Autodesk Fusion 360 part; units mm, degrees
(part 2 of 3)
sketch "Sketch5" plane through (0, 5.5, 0) normal (0, 1, 0) x (-1, 0, 0)
  line L0 (0, 36) -> (-36, 36)
  line L1 (-36, 36) -> (-36, 0)
  line L2 (-36, 0) -> (0, 0)
  line L3 (0, 0) -> (0, 36)
  circle A0 centre (-33.25, 2.75) radius 1.5
  circle A1 centre (-33.25, 33.25) radius 1.5
  circle A2 centre (-2.75, 2.75) radius 1.5
  circle A3 centre (-2.75, 33.25) radius 1.5
  line L4 (-31, 32) -> (-31, 35)
  line L5 (-31, 35) -> (-29, 35)
  line L6 (-29, 35) -> (-29, 32)
  line L7 (-29, 32) -> (-31, 32)
  line L8 (-31, 27.5714) -> (-31, 30.5714)
  line L9 (-31, 30.5714) -> (-29, 30.5714)
  line L10 (-29, 30.5714) -> (-29, 27.5714)
  line L11 (-29, 27.5714) -> (-31, 27.5714)
  line L12 (-31, 23.1429) -> (-31, 26.1429)
  line L13 (-31, 26.1429) -> (-29, 26.1429)
  line L14 (-29, 26.1429) -> (-29, 23.1429)
  line L15 (-29, 23.1429) -> (-31, 23.1429)
  line L16 (-31, 18.7143) -> (-31, 21.7143)
  line L17 (-31, 21.7143) -> (-29, 21.7143)
  line L18 (-29, 21.7143) -> (-29, 18.7143)
  line L19 (-29, 18.7143) -> (-31, 18.7143)
  line L20 (-31, 14.2857) -> (-31, 17.2857)
  line L21 (-31, 17.2857) -> (-29, 17.2857)
  line L22 (-29, 17.2857) -> (-29, 14.2857)
  line L23 (-29, 14.2857) -> (-31, 14.2857)
  line L24 (-31, 9.8571) -> (-31, 12.8571)
  line L25 (-31, 12.8571) -> (-29, 12.8571)
  line L26 (-29, 12.8571) -> (-29, 9.8571)
  line L27 (-29, 9.8571) -> (-31, 9.8571)
  line L28 (-31, 5.4286) -> (-31, 8.4286)
  line L29 (-31, 8.4286) -> (-29, 8.4286)
  line L30 (-29, 8.4286) -> (-29, 5.4286)
  line L31 (-29, 5.4286) -> (-31, 5.4286)
  line L32 (-31, 1) -> (-31, 4)
  line L33 (-31, 4) -> (-29, 4)
  line L34 (-29, 4) -> (-29, 1)
  line L35 (-29, 1) -> (-31, 1)
  line L36 (-27, 32) -> (-27, 35)
  line L37 (-27, 35) -> (-25, 35)
  line L38 (-25, 35) -> (-25, 32)
  line L39 (-25, 32) -> (-27, 32)
  line L40 (-27, 27.5714) -> (-27, 30.5714)
  line L41 (-27, 30.5714) -> (-25, 30.5714)
  line L42 (-25, 30.5714) -> (-25, 27.5714)
  line L43 (-25, 27.5714) -> (-27, 27.5714)
  line L44 (-27, 23.1429) -> (-27, 26.1429)
  line L45 (-27, 26.1429) -> (-25, 26.1429)
  line L46 (-25, 26.1429) -> (-25, 23.1429)
  line L47 (-25, 23.1429) -> (-27, 23.1429)
  line L48 (-27, 18.7143) -> (-27, 21.7143)
  line L49 (-27, 21.7143) -> (-25, 21.7143)
  line L50 (-25, 21.7143) -> (-25, 18.7143)
  line L51 (-25, 18.7143) -> (-27, 18.7143)
  line L52 (-27, 14.2857) -> (-27, 17.2857)
  line L53 (-27, 17.2857) -> (-25, 17.2857)
  line L54 (-25, 17.2857) -> (-25, 14.2857)
  line L55 (-25, 14.2857) -> (-27, 14.2857)
  line L56 (-27, 9.8571) -> (-27, 12.8571)
  line L57 (-27, 12.8571) -> (-25, 12.8571)
  line L58 (-25, 12.8571) -> (-25, 9.8571)
  line L59 (-25, 9.8571) -> (-27, 9.8571)
  line L60 (-27, 5.4286) -> (-27, 8.4286)
  line L61 (-27, 8.4286) -> (-25, 8.4286)
  line L62 (-25, 8.4286) -> (-25, 5.4286)
  line L63 (-25, 5.4286) -> (-27, 5.4286)
  line L64 (-27, 1) -> (-27, 4)
  line L65 (-27, 4) -> (-25, 4)
  line L66 (-25, 4) -> (-25, 1)
  line L67 (-25, 1) -> (-27, 1)
  line L68 (-23, 32) -> (-23, 35)
  line L69 (-23, 35) -> (-21, 35)
  line L70 (-21, 35) -> (-21, 32)
  line L71 (-21, 32) -> (-23, 32)
  line L72 (-23, 27.5714) -> (-23, 30.5714)
  line L73 (-23, 30.5714) -> (-21, 30.5714)
  line L74 (-21, 30.5714) -> (-21, 27.5714)
  line L75 (-21, 27.5714) -> (-23, 27.5714)
  line L76 (-23, 23.1429) -> (-23, 26.1429)
  line L77 (-23, 26.1429) -> (-21, 26.1429)
  line L78 (-21, 26.1429) -> (-21, 23.1429)
  line L79 (-21, 23.1429) -> (-23, 23.1429)
  line L80 (-23, 18.7143) -> (-23, 21.7143)
  line L81 (-23, 21.7143) -> (-21, 21.7143)
  line L82 (-21, 21.7143) -> (-21, 18.7143)
  line L83 (-21, 18.7143) -> (-23, 18.7143)
  line L84 (-23, 14.2857) -> (-23, 17.2857)
  line L85 (-23, 17.2857) -> (-21, 17.2857)
  line L86 (-21, 17.2857) -> (-21, 14.2857)
  line L87 (-21, 14.2857) -> (-23, 14.2857)
  line L88 (-23, 9.8571) -> (-23, 12.8571)
  line L89 (-23, 12.8571) -> (-21, 12.8571)
  line L90 (-21, 12.8571) -> (-21, 9.8571)
  line L91 (-21, 9.8571) -> (-23, 9.8571)
  line L92 (-23, 5.4286) -> (-23, 8.4286)
  line L93 (-23, 8.4286) -> (-21, 8.4286)
  line L94 (-21, 8.4286) -> (-21, 5.4286)
  line L95 (-21, 5.4286) -> (-23, 5.4286)
  line L96 (-23, 1) -> (-23, 4)
  line L97 (-23, 4) -> (-21, 4)
  line L98 (-21, 4) -> (-21, 1)
  line L99 (-21, 1) -> (-23, 1)
  line L100 (-19, 32) -> (-19, 35)
  line L101 (-19, 35) -> (-17, 35)
  line L102 (-17, 35) -> (-17, 32)
  line L103 (-17, 32) -> (-19, 32)
  line L104 (-19, 27.5714) -> (-19, 30.5714)
  line L105 (-19, 30.5714) -> (-17, 30.5714)
  line L106 (-17, 30.5714) -> (-17, 27.5714)
  line L107 (-17, 27.5714) -> (-19, 27.5714)
  line L108 (-19, 23.1429) -> (-19, 26.1429)
  line L109 (-19, 26.1429) -> (-17, 26.1429)
  line L110 (-17, 26.1429) -> (-17, 23.1429)
  line L111 (-17, 23.1429) -> (-19, 23.1429)
  line L112 (-19, 18.7143) -> (-19, 21.7143)
  line L113 (-19, 21.7143) -> (-17, 21.7143)
  line L114 (-17, 21.7143) -> (-17, 18.7143)
  line L115 (-17, 18.7143) -> (-19, 18.7143)
  line L116 (-19, 14.2857) -> (-19, 17.2857)
  line L117 (-19, 17.2857) -> (-17, 17.2857)
  line L118 (-17, 17.2857) -> (-17, 14.2857)
  line L119 (-17, 14.2857) -> (-19, 14.2857)
  line L120 (-19, 9.8571) -> (-19, 12.8571)
  line L121 (-19, 12.8571) -> (-17, 12.8571)
  line L122 (-17, 12.8571) -> (-17, 9.8571)
  line L123 (-17, 9.8571) -> (-19, 9.8571)
  line L124 (-19, 5.4286) -> (-19, 8.4286)
  line L125 (-19, 8.4286) -> (-17, 8.4286)
  line L126 (-17, 8.4286) -> (-17, 5.4286)
  line L127 (-17, 5.4286) -> (-19, 5.4286)
  line L128 (-19, 1) -> (-19, 4)
  line L129 (-19, 4) -> (-17, 4)
  line L130 (-17, 4) -> (-17, 1)
  line L131 (-17, 1) -> (-19, 1)
  line L132 (-15, 32) -> (-15, 35)
  line L133 (-15, 35) -> (-13, 35)
  line L134 (-13, 35) -> (-13, 32)
  line L135 (-13, 32) -> (-15, 32)
  line L136 (-15, 27.5714) -> (-15, 30.5714)
  line L137 (-15, 30.5714) -> (-13, 30.5714)
  line L138 (-13, 30.5714) -> (-13, 27.5714)
  line L139 (-13, 27.5714) -> (-15, 27.5714)
  line L140 (-15, 23.1429) -> (-15, 26.1429)
  line L141 (-15, 26.1429) -> (-13, 26.1429)
  line L142 (-13, 26.1429) -> (-13, 23.1429)
  line L143 (-13, 23.1429) -> (-15, 23.1429)
  line L144 (-15, 18.7143) -> (-15, 21.7143)
  line L145 (-15, 21.7143) -> (-13, 21.7143)
  line L146 (-13, 21.7143) -> (-13, 18.7143)
  line L147 (-13, 18.7143) -> (-15, 18.7143)
  line L148 (-15, 14.2857) -> (-15, 17.2857)
  line L149 (-15, 17.2857) -> (-13, 17.2857)
  line L150 (-13, 17.2857) -> (-13, 14.2857)
  line L151 (-13, 14.2857) -> (-15, 14.2857)
  line L152 (-15, 9.8571) -> (-15, 12.8571)
  line L153 (-15, 12.8571) -> (-13, 12.8571)
  line L154 (-13, 12.8571) -> (-13, 9.8571)
  line L155 (-13, 9.8571) -> (-15, 9.8571)
  line L156 (-15, 5.4286) -> (-15, 8.4286)
  line L157 (-15, 8.4286) -> (-13, 8.4286)
  line L158 (-13, 8.4286) -> (-13, 5.4286)
  line L159 (-13, 5.4286) -> (-15, 5.4286)
  line L160 (-15, 1) -> (-15, 4)
  line L161 (-15, 4) -> (-13, 4)
  line L162 (-13, 4) -> (-13, 1)
  line L163 (-13, 1) -> (-15, 1)
  line L164 (-11, 32) -> (-11, 35)
  line L165 (-11, 35) -> (-9, 35)
  line L166 (-9, 35) -> (-9, 32)
  line L167 (-9, 32) -> (-11, 32)
  line L168 (-11, 27.5714) -> (-11, 30.5714)
  line L169 (-11, 30.5714) -> (-9, 30.5714)
  line L170 (-9, 30.5714) -> (-9, 27.5714)
  line L171 (-9, 27.5714) -> (-11, 27.5714)
  line L172 (-11, 23.1429) -> (-11, 26.1429)
  line L173 (-11, 26.1429) -> (-9, 26.1429)
  line L174 (-9, 26.1429) -> (-9, 23.1429)
  line L175 (-9, 23.1429) -> (-11, 23.1429)
  line L176 (-11, 18.7143) -> (-11, 21.7143)
  line L177 (-11, 21.7143) -> (-9, 21.7143)
  line L178 (-9, 21.7143) -> (-9, 18.7143)
  line L179 (-9, 18.7143) -> (-11, 18.7143)
  line L180 (-11, 14.2857) -> (-11, 17.2857)
  line L181 (-11, 17.2857) -> (-9, 17.2857)
  line L182 (-9, 17.2857) -> (-9, 14.2857)
  line L183 (-9, 14.2857) -> (-11, 14.2857)
  line L184 (-11, 9.8571) -> (-11, 12.8571)
  line L185 (-11, 12.8571) -> (-9, 12.8571)
  line L186 (-9, 12.8571) -> (-9, 9.8571)
  line L187 (-9, 9.8571) -> (-11, 9.8571)
  line L188 (-11, 5.4286) -> (-11, 8.4286)
  line L189 (-11, 8.4286) -> (-9, 8.4286)
  line L190 (-9, 8.4286) -> (-9, 5.4286)
  line L191 (-9, 5.4286) -> (-11, 5.4286)
  line L192 (-11, 1) -> (-11, 4)
  line L193 (-11, 4) -> (-9, 4)
  line L194 (-9, 4) -> (-9, 1)
  line L195 (-9, 1) -> (-11, 1)
  line L196 (-7, 32) -> (-7, 35)
  line L197 (-7, 35) -> (-5, 35)
  line L198 (-5, 35) -> (-5, 32)
  line L199 (-5, 32) -> (-7, 32)
  line L200 (-7, 27.5714) -> (-7, 30.5714)
  line L201 (-7, 30.5714) -> (-5, 30.5714)
  line L202 (-5, 30.5714) -> (-5, 27.5714)
  line L203 (-5, 27.5714) -> (-7, 27.5714)
  line L204 (-7, 23.1429) -> (-7, 26.1429)
  line L205 (-7, 26.1429) -> (-5, 26.1429)
  line L206 (-5, 26.1429) -> (-5, 23.1429)
  line L207 (-5, 23.1429) -> (-7, 23.1429)
  line L208 (-7, 18.7143) -> (-7, 21.7143)
  line L209 (-7, 21.7143) -> (-5, 21.7143)
  line L210 (-5, 21.7143) -> (-5, 18.7143)
  line L211 (-5, 18.7143) -> (-7, 18.7143)
  line L212 (-7, 14.2857) -> (-7, 17.2857)
  line L213 (-7, 17.2857) -> (-5, 17.2857)
  line L214 (-5, 17.2857) -> (-5, 14.2857)
  line L215 (-5, 14.2857) -> (-7, 14.2857)
  line L216 (-7, 9.8571) -> (-7, 12.8571)
  line L217 (-7, 12.8571) -> (-5, 12.8571)
  line L218 (-5, 12.8571) -> (-5, 9.8571)
  line L219 (-5, 9.8571) -> (-7, 9.8571)
  line L220 (-7, 5.4286) -> (-7, 8.4286)
  line L221 (-7, 8.4286) -> (-5, 8.4286)
  line L222 (-5, 8.4286) -> (-5, 5.4286)
  line L223 (-5, 5.4286) -> (-7, 5.4286)
  line L224 (-7, 1) -> (-7, 4)
  line L225 (-7, 4) -> (-5, 4)
  line L226 (-5, 4) -> (-5, 1)
  line L227 (-5, 1) -> (-7, 1)
  line L228 (-4, 31) -> (0.3, 31)
  line L229 (0.3, 31) -> (-4, 31)
  line L230 (-4, 31) -> (-4, 5)
  line L231 (-4, 5) -> (0.5, 5)
  constraint perpendicular L3 L228
  constraint perpendicular L219 L230
  constraint perpendicular L3 L231
extrude "Extrude5" cut sketch "Sketch5" against normal blind 15 contours L3 L228 L229 L230 L231
sketch "Sketch6" plane through (0, 5.5, 0) normal (0, 1, 0) x (-1, 0, 0)
  line L0 (-7, 1) -> (-7, 4)
  line L1 (-7, 4) -> (-5, 4)
  line L2 (-5, 4) -> (-5, 1)
  line L3 (-5, 1) -> (-7, 1)
  line L4 (-7, 5.4286) -> (-7, 8.4286)
  line L5 (-7, 8.4286) -> (-5, 8.4286)
  line L6 (-5, 8.4286) -> (-5, 5.4286)
  line L7 (-5, 5.4286) -> (-7, 5.4286)
  line L8 (-7, 9.8571) -> (-7, 12.8571)
  line L9 (-7, 12.8571) -> (-5, 12.8571)
  line L10 (-5, 12.8571) -> (-5, 9.8571)
  line L11 (-5, 9.8571) -> (-7, 9.8571)
  line L12 (-7, 14.2857) -> (-7, 17.2857)
  line L13 (-7, 17.2857) -> (-5, 17.2857)
  line L14 (-5, 17.2857) -> (-5, 14.2857)
  line L15 (-5, 14.2857) -> (-7, 14.2857)
  line L16 (-7, 18.7143) -> (-7, 21.7143)
  line L17 (-7, 21.7143) -> (-5, 21.7143)
  line L18 (-5, 21.7143) -> (-5, 18.7143)
  line L19 (-5, 18.7143) -> (-7, 18.7143)
  line L20 (-7, 23.1429) -> (-7, 26.1429)
  line L21 (-7, 26.1429) -> (-5, 26.1429)
  line L22 (-5, 26.1429) -> (-5, 23.1429)
  line L23 (-5, 23.1429) -> (-7, 23.1429)
  line L24 (-7, 27.5714) -> (-7, 30.5714)
  line L25 (-7, 30.5714) -> (-5, 30.5714)
  line L26 (-5, 30.5714) -> (-5, 27.5714)
  line L27 (-5, 27.5714) -> (-7, 27.5714)
  line L28 (-7, 32) -> (-7, 35)
  line L29 (-7, 35) -> (-5, 35)
  line L30 (-5, 35) -> (-5, 32)
  line L31 (-5, 32) -> (-7, 32)
  line L32 (-11, 1) -> (-11, 4)
  line L33 (-11, 4) -> (-9, 4)
  line L34 (-9, 4) -> (-9, 1)
  line L35 (-9, 1) -> (-11, 1)
  line L36 (-11, 5.4286) -> (-11, 8.4286)
  line L37 (-11, 8.4286) -> (-9, 8.4286)
  line L38 (-9, 8.4286) -> (-9, 5.4286)
  line L39 (-9, 5.4286) -> (-11, 5.4286)
  line L40 (-11, 9.8571) -> (-11, 12.8571)
  line L41 (-11, 12.8571) -> (-9, 12.8571)
  line L42 (-9, 12.8571) -> (-9, 9.8571)
  line L43 (-9, 9.8571) -> (-11, 9.8571)
  line L44 (-11, 14.2857) -> (-11, 17.2857)
  line L45 (-11, 17.2857) -> (-9, 17.2857)
  line L46 (-9, 17.2857) -> (-9, 14.2857)
  line L47 (-9, 14.2857) -> (-11, 14.2857)
  line L48 (-11, 18.7143) -> (-11, 21.7143)
  line L49 (-11, 21.7143) -> (-9, 21.7143)
  line L50 (-9, 21.7143) -> (-9, 18.7143)
  line L51 (-9, 18.7143) -> (-11, 18.7143)
  line L52 (-11, 23.1429) -> (-11, 26.1429)
  line L53 (-11, 26.1429) -> (-9, 26.1429)
  line L54 (-9, 26.1429) -> (-9, 23.1429)
  line L55 (-9, 23.1429) -> (-11, 23.1429)
  line L56 (-11, 27.5714) -> (-11, 30.5714)
  line L57 (-11, 30.5714) -> (-9, 30.5714)
  line L58 (-9, 30.5714) -> (-9, 27.5714)
  line L59 (-9, 27.5714) -> (-11, 27.5714)
  line L60 (-11, 32) -> (-11, 35)
  line L61 (-11, 35) -> (-9, 35)
  line L62 (-9, 35) -> (-9, 32)
  line L63 (-9, 32) -> (-11, 32)
  line L64 (-15, 1) -> (-15, 4)
  line L65 (-15, 4) -> (-13, 4)
  line L66 (-13, 4) -> (-13, 1)
  line L67 (-13, 1) -> (-15, 1)
  line L68 (-15, 5.4286) -> (-15, 8.4286)
  line L69 (-15, 8.4286) -> (-13, 8.4286)
  line L70 (-13, 8.4286) -> (-13, 5.4286)
  line L71 (-13, 5.4286) -> (-15, 5.4286)
  line L72 (-15, 9.8571) -> (-15, 12.8571)
  line L73 (-15, 12.8571) -> (-13, 12.8571)
  line L74 (-13, 12.8571) -> (-13, 9.8571)
  line L75 (-13, 9.8571) -> (-15, 9.8571)
  line L76 (-15, 14.2857) -> (-15, 17.2857)
  line L77 (-15, 17.2857) -> (-13, 17.2857)
  line L78 (-13, 17.2857) -> (-13, 14.2857)
  line L79 (-13, 14.2857) -> (-15, 14.2857)
  line L80 (-15, 18.7143) -> (-15, 21.7143)
  line L81 (-15, 21.7143) -> (-13, 21.7143)
  line L82 (-13, 21.7143) -> (-13, 18.7143)
  line L83 (-13, 18.7143) -> (-15, 18.7143)
  line L84 (-15, 23.1429) -> (-15, 26.1429)
  line L85 (-15, 26.1429) -> (-13, 26.1429)
  line L86 (-13, 26.1429) -> (-13, 23.1429)
  line L87 (-13, 23.1429) -> (-15, 23.1429)
  line L88 (-15, 27.5714) -> (-15, 30.5714)
  line L89 (-15, 30.5714) -> (-13, 30.5714)
  line L90 (-13, 30.5714) -> (-13, 27.5714)
  line L91 (-13, 27.5714) -> (-15, 27.5714)
  line L92 (-15, 32) -> (-15, 35)
  line L93 (-15, 35) -> (-13, 35)
  line L94 (-13, 35) -> (-13, 32)
  line L95 (-13, 32) -> (-15, 32)
  line L96 (-19, 1) -> (-19, 4)
  line L97 (-19, 4) -> (-17, 4)
  line L98 (-17, 4) -> (-17, 1)
  line L99 (-17, 1) -> (-19, 1)
  line L100 (-19, 5.4286) -> (-19, 8.4286)
  line L101 (-19, 8.4286) -> (-17, 8.4286)
  line L102 (-17, 8.4286) -> (-17, 5.4286)
  line L103 (-17, 5.4286) -> (-19, 5.4286)
  line L104 (-19, 9.8571) -> (-19, 12.8571)
  line L105 (-19, 12.8571) -> (-17, 12.8571)
  line L106 (-17, 12.8571) -> (-17, 9.8571)
  line L107 (-17, 9.8571) -> (-19, 9.8571)
  line L108 (-19, 14.2857) -> (-19, 17.2857)
  line L109 (-19, 17.2857) -> (-17, 17.2857)
  line L110 (-17, 17.2857) -> (-17, 14.2857)
  line L111 (-17, 14.2857) -> (-19, 14.2857)
  line L112 (-19, 18.7143) -> (-19, 21.7143)
  line L113 (-19, 21.7143) -> (-17, 21.7143)
  line L114 (-17, 21.7143) -> (-17, 18.7143)
  line L115 (-17, 18.7143) -> (-19, 18.7143)
  line L116 (-19, 23.1429) -> (-19, 26.1429)
  line L117 (-19, 26.1429) -> (-17, 26.1429)
  line L118 (-17, 26.1429) -> (-17, 23.1429)
  line L119 (-17, 23.1429) -> (-19, 23.1429)
  line L120 (-19, 27.5714) -> (-19, 30.5714)
  line L121 (-19, 30.5714) -> (-17, 30.5714)
  line L122 (-17, 30.5714) -> (-17, 27.5714)
  line L123 (-17, 27.5714) -> (-19, 27.5714)
  line L124 (-19, 32) -> (-19, 35)
  line L125 (-19, 35) -> (-17, 35)
  line L126 (-17, 35) -> (-17, 32)
  line L127 (-17, 32) -> (-19, 32)
  line L128 (-23, 1) -> (-23, 4)
  line L129 (-23, 4) -> (-21, 4)
  line L130 (-21, 4) -> (-21, 1)
  line L131 (-21, 1) -> (-23, 1)
  line L132 (-23, 5.4286) -> (-23, 8.4286)
  line L133 (-23, 8.4286) -> (-21, 8.4286)
  line L134 (-21, 8.4286) -> (-21, 5.4286)
  line L135 (-21, 5.4286) -> (-23, 5.4286)
  line L136 (-23, 9.8571) -> (-23, 12.8571)
  line L137 (-23, 12.8571) -> (-21, 12.8571)
  line L138 (-21, 12.8571) -> (-21, 9.8571)
  line L139 (-21, 9.8571) -> (-23, 9.8571)
  line L140 (-23, 14.2857) -> (-23, 17.2857)
  line L141 (-23, 17.2857) -> (-21, 17.2857)
  line L142 (-21, 17.2857) -> (-21, 14.2857)
  line L143 (-21, 14.2857) -> (-23, 14.2857)
  line L144 (-23, 18.7143) -> (-23, 21.7143)
  line L145 (-23, 21.7143) -> (-21, 21.7143)
  line L146 (-21, 21.7143) -> (-21, 18.7143)
  line L147 (-21, 18.7143) -> (-23, 18.7143)
  line L148 (-23, 23.1429) -> (-23, 26.1429)
  line L149 (-23, 26.1429) -> (-21, 26.1429)
  line L150 (-21, 26.1429) -> (-21, 23.1429)
  line L151 (-21, 23.1429) -> (-23, 23.1429)
  line L152 (-23, 27.5714) -> (-23, 30.5714)
  line L153 (-23, 30.5714) -> (-21, 30.5714)
  line L154 (-21, 30.5714) -> (-21, 27.5714)
  line L155 (-21, 27.5714) -> (-23, 27.5714)
  line L156 (-23, 32) -> (-23, 35)
  line L157 (-23, 35) -> (-21, 35)
  line L158 (-21, 35) -> (-21, 32)
  line L159 (-21, 32) -> (-23, 32)
  line L160 (-27, 1) -> (-27, 4)
  line L161 (-27, 4) -> (-25, 4)
  line L162 (-25, 4) -> (-25, 1)
  line L163 (-25, 1) -> (-27, 1)
  line L164 (-27, 5.4286) -> (-27, 8.4286)
  line L165 (-27, 8.4286) -> (-25, 8.4286)
  line L166 (-25, 8.4286) -> (-25, 5.4286)
  line L167 (-25, 5.4286) -> (-27, 5.4286)
  line L168 (-27, 9.8571) -> (-27, 12.8571)
  line L169 (-27, 12.8571) -> (-25, 12.8571)
  line L170 (-25, 12.8571) -> (-25, 9.8571)
  line L171 (-25, 9.8571) -> (-27, 9.8571)
  line L172 (-27, 14.2857) -> (-27, 17.2857)
  line L173 (-27, 17.2857) -> (-25, 17.2857)
  line L174 (-25, 17.2857) -> (-25, 14.2857)
  line L175 (-25, 14.2857) -> (-27, 14.2857)
  line L176 (-27, 18.7143) -> (-27, 21.7143)
  line L177 (-27, 21.7143) -> (-25, 21.7143)
  line L178 (-25, 21.7143) -> (-25, 18.7143)
  line L179 (-25, 18.7143) -> (-27, 18.7143)
  line L180 (-27, 23.1429) -> (-27, 26.1429)
  line L181 (-27, 26.1429) -> (-25, 26.1429)
  line L182 (-25, 26.1429) -> (-25, 23.1429)
  line L183 (-25, 23.1429) -> (-27, 23.1429)
  line L184 (-27, 27.5714) -> (-27, 30.5714)
  line L185 (-27, 30.5714) -> (-25, 30.5714)
  line L186 (-25, 30.5714) -> (-25, 27.5714)
  line L187 (-25, 27.5714) -> (-27, 27.5714)
  line L188 (-27, 32) -> (-27, 35)
  line L189 (-27, 35) -> (-25, 35)
  line L190 (-25, 35) -> (-25, 32)
  line L191 (-25, 32) -> (-27, 32)
  line L192 (-31, 1) -> (-31, 4)
  line L193 (-31, 4) -> (-29, 4)
  line L194 (-29, 4) -> (-29, 1)
  line L195 (-29, 1) -> (-31, 1)
  line L196 (-31, 5.4286) -> (-31, 8.4286)
  line L197 (-31, 8.4286) -> (-29, 8.4286)
  line L198 (-29, 8.4286) -> (-29, 5.4286)
  line L199 (-29, 5.4286) -> (-31, 5.4286)
  line L200 (-31, 9.8571) -> (-31, 12.8571)
  line L201 (-31, 12.8571) -> (-29, 12.8571)
  line L202 (-29, 12.8571) -> (-29, 9.8571)
  line L203 (-29, 9.8571) -> (-31, 9.8571)
  line L204 (-31, 14.2857) -> (-31, 17.2857)
  line L205 (-31, 17.2857) -> (-29, 17.2857)
  line L206 (-29, 17.2857) -> (-29, 14.2857)
  line L207 (-29, 14.2857) -> (-31, 14.2857)
  line L208 (-31, 18.7143) -> (-31, 21.7143)
  line L209 (-31, 21.7143) -> (-29, 21.7143)
  line L210 (-29, 21.7143) -> (-29, 18.7143)
  line L211 (-29, 18.7143) -> (-31, 18.7143)
  line L212 (-31, 23.1429) -> (-31, 26.1429)
  line L213 (-31, 26.1429) -> (-29, 26.1429)
  line L214 (-29, 26.1429) -> (-29, 23.1429)
  line L215 (-29, 23.1429) -> (-31, 23.1429)
  line L216 (-31, 27.5714) -> (-31, 30.5714)
  line L217 (-31, 30.5714) -> (-29, 30.5714)
  line L218 (-29, 30.5714) -> (-29, 27.5714)
  line L219 (-29, 27.5714) -> (-31, 27.5714)
  line L220 (-31, 32) -> (-31, 35)
  line L221 (-31, 35) -> (-29, 35)
  line L222 (-29, 35) -> (-29, 32)
  line L223 (-29, 32) -> (-31, 32)
  circle A0 centre (-2.75, 33.25) radius 1.5
  circle A1 centre (-2.75, 2.75) radius 1.5
  circle A2 centre (-33.25, 33.25) radius 1.5
  circle A3 centre (-33.25, 2.75) radius 1.5
  line L224 (-4, 31) -> (0, 31)
  line L225 (0, 31) -> (0, 36)
  line L226 (0, 36) -> (-36, 36)
  line L227 (-36, 36) -> (-36, 0)
  line L228 (-36, 0) -> (0, 0)
  line L229 (0, 0) -> (0, 5)
  line L230 (0, 5) -> (-4, 5)
  line L231 (-4, 5) -> (-4, 31)
  line L232 (-36, 31) -> (-32, 31)
  line L233 (-32, 31) -> (-32, 5)
  line L234 (-32, 5) -> (-36, 5)
  constraint coincident L227 L232.start
  constraint perpendicular L227 L232
  constraint perpendicular L199 L233
  constraint coincident L227 L234.end
  constraint perpendicular L227 L234
extrude "Extrude6" cut sketch "Sketch6" against normal blind 15 contours L227 L232 L233 L234
sketch "Sketch7" plane through (0, 0, 36) normal (0, 0, 1) x (-1, 0, 0)
  line L0 (0, 0) -> (-36, 0)
  line L1 (-36, 0) -> (-36, -5.5)
  line L2 (-36, -5.5) -> (0, -5.5)
  line L3 (0, -5.5) -> (0, 0)
  circle A0 centre (-18, -2.75) radius 2.5
  dimension "d32" = 5
  measures "d32" diameter of A0
extrude "Extrude7" add sketch "Sketch7" along normal blind 3 contours A0
sketch "Sketch8" plane through (0, 0, 0) normal (0, -1, 0) x (1, 0, 0)
  line L0 (32, 31) -> (36, 31)
  line L1 (36, 31) -> (36, 36)
  line L2 (36, 36) -> (0, 36)
  line L3 (0, 36) -> (0, 31)
  line L4 (0, 31) -> (4, 31)
  line L5 (4, 31) -> (4, 5)
  line L6 (4, 5) -> (0, 5)
  line L7 (0, 5) -> (0, 0)
  line L8 (0, 0) -> (36, 0)
  line L9 (36, 0) -> (36, 5)
  line L10 (36, 5) -> (32, 5)
  line L11 (32, 5) -> (32, 31)
  circle A0 centre (33.25, 2.75) radius 1.5
  circle A1 centre (33.25, 33.25) radius 1.5
  circle A2 centre (2.75, 2.75) radius 1.5
  circle A3 centre (2.75, 33.25) radius 1.5
  line L12 (31, 18) -> (29, 18)
  line L13 (29, 18) -> (29, 28)
  line L14 (29, 28) -> (31, 28)
  line L15 (31, 28) -> (31, 18)
  line L16 (29.2903, 27.5521) -> (30.7537, 27.5521)
  line L17 (30.7537, 27.5521) -> (30.7537, 25.0331)
  line L18 (30.7537, 25.0331) -> (29.2903, 25.0331)
  line L19 (29.2903, 25.0331) -> (29.2903, 27.5521)
  line L20 (29.2903, 24.3827) -> (30.7537, 24.3827)
  line L21 (30.7537, 24.3827) -> (30.7537, 21.7556)
  line L22 (30.7537, 21.7556) -> (29.2903, 21.7556)
  line L23 (29.2903, 21.7556) -> (29.2903, 24.3827)
  line L24 (29.2903, 21.0379) -> (30.7537, 21.0379)
  line L25 (30.7537, 21.0379) -> (30.7537, 18.3132)
  line L26 (30.7537, 18.3132) -> (29.2903, 18.3132)
  line L27 (29.2903, 18.3132) -> (29.2903, 21.0379)
  constraint horizontal L12
  constraint vertical L13
  constraint horizontal L14
  constraint vertical L15
  constraint horizontal L16
  constraint vertical L17
  constraint horizontal L18
  constraint vertical L19
  constraint horizontal L20
  constraint vertical L21
  constraint horizontal L22
  constraint vertical L23
  constraint horizontal L24
  constraint vertical L25
  constraint horizontal L26
  constraint vertical L27
extrude "Extrude8" add sketch "Sketch8" along normal blind 1 contours L16 L17 L18 L19 | L20 L21 L22 L23 | L24 L25 L26 L27
sketch "Sketch9" plane through (32, 0, 0) normal (1, 0, 0) x (0, 1, 0)
  line L0 (0, 31) -> (0, 5)
  line L1 (0, 5) -> (5.5, 5)
  line L2 (5.5, 5) -> (5.5, 31)
  line L3 (5.5, 31) -> (0, 31)
  line L4 (2, 12.9249) -> (3.5, 12.9249)
  line L5 (3.5, 12.9249) -> (3.5, 10)
  line L6 (3.5, 10) -> (2, 10)
  line L7 (2, 10) -> (2, 12.9249)
  constraint horizontal L4
  constraint vertical L5
  constraint horizontal L6
  constraint vertical L7
extrude "Extrude9" add sketch "Sketch9" along normal blind 1 contours L4 L5 L6 L7
sketch "Sketch10" plane through (0, 0, 0) normal (0, -1, 0) x (1, 0, 0)
  line L0 (29.2903, 25.0331) -> (29.2903, 27.5521)
  line L1 (29.2903, 27.5521) -> (30.7537, 27.5521)
  line L2 (30.7537, 27.5521) -> (30.7537, 25.0331)
  line L3 (30.7537, 25.0331) -> (29.2903, 25.0331)
  line L4 (29.2903, 21.7556) -> (29.2903, 24.3827)
  line L5 (29.2903, 24.3827) -> (30.7537, 24.3827)
  line L6 (30.7537, 24.3827) -> (30.7537, 21.7556)
  line L7 (30.7537, 21.7556) -> (29.2903, 21.7556)
  line L8 (29.2903, 18.3132) -> (29.2903, 21.0379)
  line L9 (29.2903, 21.0379) -> (30.7537, 21.0379)
  line L10 (30.7537, 21.0379) -> (30.7537, 18.3132)
  line L11 (30.7537, 18.3132) -> (29.2903, 18.3132)
  line L12 (32, 31) -> (36, 31)
  line L13 (36, 31) -> (36, 36)
  line L14 (36, 36) -> (0, 36)
  line L15 (0, 36) -> (0, 31)
  line L16 (0, 31) -> (4, 31)
  line L17 (4, 31) -> (4, 5)
  line L18 (4, 5) -> (0, 5)
  line L19 (0, 5) -> (0, 0)
  line L20 (0, 0) -> (36, 0)
  line L21 (36, 0) -> (36, 5)
  line L22 (36, 5) -> (32, 5)
  line L23 (32, 5) -> (32, 31)
  circle A0 centre (33.25, 2.75) radius 1.5
  circle A1 centre (33.25, 33.25) radius 1.5
  circle A2 centre (2.75, 2.75) radius 1.5
  circle A3 centre (2.75, 33.25) radius 1.5
  line L24 (5.0897, 18.3132) -> (12, 18.3132)
  line L25 (12, 18.3132) -> (12, 11)
  line L26 (12, 11) -> (5.0897, 11)
  line L27 (5.0897, 11) -> (5.0897, 18.3132)
  constraint horizontal L24
  constraint vertical L25
  constraint horizontal L26
  constraint vertical L27
extrude "Extrude10" add sketch "Sketch10" along normal blind 1 contours L24 L25 L26 L27
sketch "Sketch11" plane through (0, 0, 0) normal (0, -1, 0) x (1, 0, 0)
  circle A0 centre (2.75, 33.25) radius 1.5
  circle A1 centre (2.75, 2.75) radius 1.5
  circle A2 centre (33.25, 33.25) radius 1.5
  circle A3 centre (33.25, 2.75) radius 1.5
  line L0 (32, 31) -> (36, 31)
  line L1 (36, 31) -> (36, 36)
  line L2 (36, 36) -> (0, 36)
  line L3 (0, 36) -> (0, 31)
  line L4 (0, 31) -> (4, 31)
  line L5 (4, 31) -> (4, 5)
  line L6 (4, 5) -> (0, 5)
  line L7 (0, 5) -> (0, 0)
  line L8 (0, 0) -> (36, 0)
  line L9 (36, 0) -> (36, 5)
  line L10 (36, 5) -> (32, 5)
  line L11 (32, 5) -> (32, 31)
  line L12 (29.2903, 18.3132) -> (29.2903, 21.0379)
  line L13 (29.2903, 21.0379) -> (30.7537, 21.0379)
  line L14 (30.7537, 21.0379) -> (30.7537, 18.3132)
  line L15 (30.7537, 18.3132) -> (29.2903, 18.3132)
  line L16 (29.2903, 21.7556) -> (29.2903, 24.3827)
  line L17 (29.2903, 24.3827) -> (30.7537, 24.3827)
  line L18 (30.7537, 24.3827) -> (30.7537, 21.7556)
  line L19 (30.7537, 21.7556) -> (29.2903, 21.7556)
  line L20 (29.2903, 25.0331) -> (29.2903, 27.5521)
  line L21 (29.2903, 27.5521) -> (30.7537, 27.5521)
  line L22 (30.7537, 27.5521) -> (30.7537, 25.0331)
  line L23 (30.7537, 25.0331) -> (29.2903, 25.0331)
  line L24 (5.0897, 11) -> (5.0897, 18.3132)
  line L25 (5.0897, 18.3132) -> (12, 18.3132)
  line L26 (12, 18.3132) -> (12, 11)
  line L27 (12, 11) -> (5.0897, 11)
  line L28 (13, 0) -> (23, 0)
  line L29 (23, 0) -> (23, 4.9683)
  line L30 (23, 4.9683) -> (13, 4.9683)
  line L31 (13, 4.9683) -> (13, 0)
  constraint horizontal L28
  constraint vertical L29
  constraint horizontal L30
  constraint vertical L31
  constraint coincident L8 L28.start
extrude "Extrude11" add sketch "Sketch11" along normal blind 1 contours L8 L28 L29 L30 L31
sketch "Sketch12" plane through (0, 0, 0) normal (0, 0, -1) x (1, 0, 0)
  line L0 (13, 0) -> (0, 0)
  line L1 (0, 0) -> (0, -5.5)
  line L2 (0, -5.5) -> (36, -5.5)
  line L3 (36, -5.5) -> (36, 0)
  line L4 (36, 0) -> (23, 0)
  line L5 (23, 0) -> (23, 1)
  line L6 (23, 1) -> (13, 1)
  line L7 (13, 1) -> (13, 0)
  line L8 (22.621, -1.0763) -> (13.4121, -1.0763)
  line L9 (13.4121, -1.0763) -> (13.4121, 0.5912)
  line L10 (13.4121, 0.5912) -> (22.621, 0.5912)
  line L11 (22.621, 0.5912) -> (22.621, -1.0763)
  constraint horizontal L8
  constraint vertical L9
  constraint horizontal L10
  constraint vertical L11
extrude "Extrude12" cut sketch "Sketch12" against normal blind 1 contours L8 L9 L10 L11
sketch "Sketch13" plane through (0, 5.5, 0) normal (0, 1, 0) x (-1, 0, 0)
  line L0 (-36, 31) -> (-32, 31)
  line L1 (-32, 31) -> (-32, 5)
  line L2 (-32, 5) -> (-36, 5)
  line L3 (-36, 5) -> (-36, 0)
  line L4 (-36, 0) -> (0, 0)
  line L5 (0, 0) -> (0, 5)
  line L6 (0, 5) -> (-4, 5)
  line L7 (-4, 5) -> (-4, 31)
  line L8 (-4, 31) -> (0, 31)
  line L9 (0, 31) -> (0, 36)
  line L10 (0, 36) -> (-36, 36)
  line L11 (-36, 36) -> (-36, 31)
  circle A0 centre (-33.25, 2.75) radius 1.5
  circle A1 centre (-33.25, 33.25) radius 1.5
  circle A2 centre (-2.75, 2.75) radius 1.5
  circle A3 centre (-2.75, 33.25) radius 1.5
  line L12 (-31, 32) -> (-31, 35)
  line L13 (-31, 35) -> (-29, 35)
  line L14 (-29, 35) -> (-29, 32)
  line L15 (-29, 32) -> (-31, 32)
  line L16 (-31, 27.5714) -> (-31, 30.5714)
  line L17 (-31, 30.5714) -> (-29, 30.5714)
  line L18 (-29, 30.5714) -> (-29, 27.5714)
  line L19 (-29, 27.5714) -> (-31, 27.5714)
  line L20 (-31, 23.1429) -> (-31, 26.1429)
  line L21 (-31, 26.1429) -> (-29, 26.1429)
  line L22 (-29, 26.1429) -> (-29, 23.1429)
  line L23 (-29, 23.1429) -> (-31, 23.1429)
  line L24 (-31, 18.7143) -> (-31, 21.7143)
  line L25 (-31, 21.7143) -> (-29, 21.7143)
  line L26 (-29, 21.7143) -> (-29, 18.7143)
  line L27 (-29, 18.7143) -> (-31, 18.7143)
  line L28 (-31, 14.2857) -> (-31, 17.2857)
  line L29 (-31, 17.2857) -> (-29, 17.2857)
  line L30 (-29, 17.2857) -> (-29, 14.2857)
  line L31 (-29, 14.2857) -> (-31, 14.2857)
  line L32 (-31, 9.8571) -> (-31, 12.8571)
  line L33 (-31, 12.8571) -> (-29, 12.8571)
  line L34 (-29, 12.8571) -> (-29, 9.8571)
  line L35 (-29, 9.8571) -> (-31, 9.8571)
  line L36 (-31, 5.4286) -> (-31, 8.4286)
  line L37 (-31, 8.4286) -> (-29, 8.4286)
  line L38 (-29, 8.4286) -> (-29, 5.4286)
  line L39 (-29, 5.4286) -> (-31, 5.4286)
  line L40 (-31, 1) -> (-31, 4)
  line L41 (-31, 4) -> (-29, 4)
  line L42 (-29, 4) -> (-29, 1)
  line L43 (-29, 1) -> (-31, 1)
  line L44 (-27, 32) -> (-27, 35)
  line L45 (-27, 35) -> (-25, 35)
  line L46 (-25, 35) -> (-25, 32)
  line L47 (-25, 32) -> (-27, 32)
  line L48 (-27, 27.5714) -> (-27, 30.5714)
  line L49 (-27, 30.5714) -> (-25, 30.5714)
  line L50 (-25, 30.5714) -> (-25, 27.5714)
  line L51 (-25, 27.5714) -> (-27, 27.5714)
  line L52 (-27, 23.1429) -> (-27, 26.1429)
  line L53 (-27, 26.1429) -> (-25, 26.1429)
  line L54 (-25, 26.1429) -> (-25, 23.1429)
  line L55 (-25, 23.1429) -> (-27, 23.1429)
  line L56 (-27, 18.7143) -> (-27, 21.7143)
  line L57 (-27, 21.7143) -> (-25, 21.7143)
  line L58 (-25, 21.7143) -> (-25, 18.7143)
  line L59 (-25, 18.7143) -> (-27, 18.7143)
  line L60 (-27, 14.2857) -> (-27, 17.2857)
  line L61 (-27, 17.2857) -> (-25, 17.2857)
  line L62 (-25, 17.2857) -> (-25, 14.2857)
  line L63 (-25, 14.2857) -> (-27, 14.2857)
  line L64 (-27, 9.8571) -> (-27, 12.8571)
  line L65 (-27, 12.8571) -> (-25, 12.8571)
  line L66 (-25, 12.8571) -> (-25, 9.8571)
  line L67 (-25, 9.8571) -> (-27, 9.8571)
  line L68 (-27, 5.4286) -> (-27, 8.4286)
  line L69 (-27, 8.4286) -> (-25, 8.4286)
  line L70 (-25, 8.4286) -> (-25, 5.4286)
  line L71 (-25, 5.4286) -> (-27, 5.4286)
  line L72 (-27, 1) -> (-27, 4)
  line L73 (-27, 4) -> (-25, 4)
  line L74 (-25, 4) -> (-25, 1)
  line L75 (-25, 1) -> (-27, 1)
  line L76 (-23, 32) -> (-23, 35)
  line L77 (-23, 35) -> (-21, 35)
  line L78 (-21, 35) -> (-21, 32)
  line L79 (-21, 32) -> (-23, 32)
  line L80 (-23, 27.5714) -> (-23, 30.5714)
  line L81 (-23, 30.5714) -> (-21, 30.5714)
  line L82 (-21, 30.5714) -> (-21, 27.5714)
  line L83 (-21, 27.5714) -> (-23, 27.5714)
  line L84 (-23, 23.1429) -> (-23, 26.1429)
  line L85 (-23, 26.1429) -> (-21, 26.1429)
  line L86 (-21, 26.1429) -> (-21, 23.1429)
  line L87 (-21, 23.1429) -> (-23, 23.1429)
  line L88 (-23, 18.7143) -> (-23, 21.7143)
  line L89 (-23, 21.7143) -> (-21, 21.7143)
  line L90 (-21, 21.7143) -> (-21, 18.7143)
  line L91 (-21, 18.7143) -> (-23, 18.7143)
  line L92 (-23, 14.2857) -> (-23, 17.2857)
  line L93 (-23, 17.2857) -> (-21, 17.2857)
  line L94 (-21, 17.2857) -> (-21, 14.2857)
  line L95 (-21, 14.2857) -> (-23, 14.2857)
  line L96 (-23, 9.8571) -> (-23, 12.8571)
  line L97 (-23, 12.8571) -> (-21, 12.8571)
  line L98 (-21, 12.8571) -> (-21, 9.8571)
  line L99 (-21, 9.8571) -> (-23, 9.8571)
  line L100 (-23, 5.4286) -> (-23, 8.4286)
  line L101 (-23, 8.4286) -> (-21, 8.4286)
  line L102 (-21, 8.4286) -> (-21, 5.4286)
  line L103 (-21, 5.4286) -> (-23, 5.4286)
  line L104 (-23, 1) -> (-23, 4)
  line L105 (-23, 4) -> (-21, 4)
  line L106 (-21, 4) -> (-21, 1)
  line L107 (-21, 1) -> (-23, 1)
  line L108 (-19, 32) -> (-19, 35)
  line L109 (-19, 35) -> (-17, 35)
  line L110 (-17, 35) -> (-17, 32)
  line L111 (-17, 32) -> (-19, 32)
  line L112 (-19, 27.5714) -> (-19, 30.5714)
  line L113 (-19, 30.5714) -> (-17, 30.5714)
  line L114 (-17, 30.5714) -> (-17, 27.5714)
  line L115 (-17, 27.5714) -> (-19, 27.5714)
  line L116 (-19, 23.1429) -> (-19, 26.1429)
  line L117 (-19, 26.1429) -> (-17, 26.1429)
  line L118 (-17, 26.1429) -> (-17, 23.1429)
  line L119 (-17, 23.1429) -> (-19, 23.1429)
  line L120 (-19, 18.7143) -> (-19, 21.7143)
  line L121 (-19, 21.7143) -> (-17, 21.7143)
  line L122 (-17, 21.7143) -> (-17, 18.7143)
  line L123 (-17, 18.7143) -> (-19, 18.7143)
  line L124 (-19, 14.2857) -> (-19, 17.2857)
  line L125 (-19, 17.2857) -> (-17, 17.2857)
  line L126 (-17, 17.2857) -> (-17, 14.2857)
  line L127 (-17, 14.2857) -> (-19, 14.2857)
  line L128 (-19, 9.8571) -> (-19, 12.8571)
  line L129 (-19, 12.8571) -> (-17, 12.8571)
  line L130 (-17, 12.8571) -> (-17, 9.8571)
  line L131 (-17, 9.8571) -> (-19, 9.8571)
  line L132 (-19, 5.4286) -> (-19, 8.4286)
  line L133 (-19, 8.4286) -> (-17, 8.4286)
  line L134 (-17, 8.4286) -> (-17, 5.4286)
  line L135 (-17, 5.4286) -> (-19, 5.4286)
  line L136 (-19, 1) -> (-19, 4)
  line L137 (-19, 4) -> (-17, 4)
  line L138 (-17, 4) -> (-17, 1)
  line L139 (-17, 1) -> (-19, 1)
  line L140 (-15, 32) -> (-15, 35)
  line L141 (-15, 35) -> (-13, 35)
  line L142 (-13, 35) -> (-13, 32)
  line L143 (-13, 32) -> (-15, 32)
  line L144 (-15, 27.5714) -> (-15, 30.5714)
  line L145 (-15, 30.5714) -> (-13, 30.5714)
  line L146 (-13, 30.5714) -> (-13, 27.5714)
  line L147 (-13, 27.5714) -> (-15, 27.5714)
  line L148 (-15, 23.1429) -> (-15, 26.1429)
  line L149 (-15, 26.1429) -> (-13, 26.1429)
  line L150 (-13, 26.1429) -> (-13, 23.1429)
  line L151 (-13, 23.1429) -> (-15, 23.1429)
  line L152 (-15, 18.7143) -> (-15, 21.7143)
  line L153 (-15, 21.7143) -> (-13, 21.7143)
  line L154 (-13, 21.7143) -> (-13, 18.7143)
  line L155 (-13, 18.7143) -> (-15, 18.7143)
  line L156 (-15, 14.2857) -> (-15, 17.2857)
  line L157 (-15, 17.2857) -> (-13, 17.2857)
  line L158 (-13, 17.2857) -> (-13, 14.2857)
  line L159 (-13, 14.2857) -> (-15, 14.2857)
  line L160 (-15, 9.8571) -> (-15, 12.8571)
  line L161 (-15, 12.8571) -> (-13, 12.8571)
  line L162 (-13, 12.8571) -> (-13, 9.8571)
  line L163 (-13, 9.8571) -> (-15, 9.8571)
  line L164 (-15, 5.4286) -> (-15, 8.4286)
  line L165 (-15, 8.4286) -> (-13, 8.4286)
  line L166 (-13, 8.4286) -> (-13, 5.4286)
  line L167 (-13, 5.4286) -> (-15, 5.4286)
  line L168 (-15, 1) -> (-15, 4)
  line L169 (-15, 4) -> (-13, 4)
  line L170 (-13, 4) -> (-13, 1)
  line L171 (-13, 1) -> (-15, 1)
  line L172 (-11, 32) -> (-11, 35)
  line L173 (-11, 35) -> (-9, 35)
  line L174 (-9, 35) -> (-9, 32)
  line L175 (-9, 32) -> (-11, 32)
  line L176 (-11, 27.5714) -> (-11, 30.5714)
  line L177 (-11, 30.5714) -> (-9, 30.5714)
  line L178 (-9, 30.5714) -> (-9, 27.5714)
  line L179 (-9, 27.5714) -> (-11, 27.5714)
  line L180 (-11, 23.1429) -> (-11, 26.1429)
  line L181 (-11, 26.1429) -> (-9, 26.1429)
  line L182 (-9, 26.1429) -> (-9, 23.1429)
  line L183 (-9, 23.1429) -> (-11, 23.1429)
  line L184 (-11, 18.7143) -> (-11, 21.7143)
  line L185 (-11, 21.7143) -> (-9, 21.7143)
  line L186 (-9, 21.7143) -> (-9, 18.7143)
  line L187 (-9, 18.7143) -> (-11, 18.7143)
  line L188 (-11, 14.2857) -> (-11, 17.2857)
  line L189 (-11, 17.2857) -> (-9, 17.2857)
  line L190 (-9, 17.2857) -> (-9, 14.2857)
  line L191 (-9, 14.2857) -> (-11, 14.2857)
  line L192 (-11, 9.8571) -> (-11, 12.8571)
  line L193 (-11, 12.8571) -> (-9, 12.8571)
  line L194 (-9, 12.8571) -> (-9, 9.8571)
  line L195 (-9, 9.8571) -> (-11, 9.8571)
  line L196 (-11, 5.4286) -> (-11, 8.4286)
  line L197 (-11, 8.4286) -> (-9, 8.4286)
  line L198 (-9, 8.4286) -> (-9, 5.4286)
  line L199 (-9, 5.4286) -> (-11, 5.4286)
  line L200 (-11, 1) -> (-11, 4)
  line L201 (-11, 4) -> (-9, 4)
  line L202 (-9, 4) -> (-9, 1)
  line L203 (-9, 1) -> (-11, 1)
  line L204 (-7, 32) -> (-7, 35)
  line L205 (-7, 35) -> (-5, 35)
  line L206 (-5, 35) -> (-5, 32)
  line L207 (-5, 32) -> (-7, 32)
  line L208 (-7, 27.5714) -> (-7, 30.5714)
  line L209 (-7, 30.5714) -> (-5, 30.5714)
  line L210 (-5, 30.5714) -> (-5, 27.5714)
  line L211 (-5, 27.5714) -> (-7, 27.5714)
  line L212 (-7, 23.1429) -> (-7, 26.1429)
  line L213 (-7, 26.1429) -> (-5, 26.1429)
  line L214 (-5, 26.1429) -> (-5, 23.1429)
  line L215 (-5, 23.1429) -> (-7, 23.1429)
  line L216 (-7, 18.7143) -> (-7, 21.7143)
  line L217 (-7, 21.7143) -> (-5, 21.7143)
  line L218 (-5, 21.7143) -> (-5, 18.7143)
  line L219 (-5, 18.7143) -> (-7, 18.7143)
  line L220 (-7, 14.2857) -> (-7, 17.2857)
  line L221 (-7, 17.2857) -> (-5, 17.2857)
  line L222 (-5, 17.2857) -> (-5, 14.2857)
  line L223 (-5, 14.2857) -> (-7, 14.2857)
  line L224 (-7, 9.8571) -> (-7, 12.8571)
  line L225 (-7, 12.8571) -> (-5, 12.8571)
  line L226 (-5, 12.8571) -> (-5, 9.8571)
  line L227 (-5, 9.8571) -> (-7, 9.8571)
  line L228 (-7, 5.4286) -> (-7, 8.4286)
  line L229 (-7, 8.4286) -> (-5, 8.4286)
  line L230 (-5, 8.4286) -> (-5, 5.4286)
  line L231 (-5, 5.4286) -> (-7, 5.4286)
  line L232 (-7, 1) -> (-7, 4)
  line L233 (-7, 4) -> (-5, 4)
  line L234 (-5, 4) -> (-5, 1)
  line L235 (-5, 1) -> (-7, 1)
  line L236 (-2.75, 2.75) -> (-33.25, 2.75)
  line L237 (-33.25, 2.75) -> (-2.75, 33.25)
  line L238 (-2.75, 33.25) -> (-33.25, 33.25)
  line L239 (-33.25, 33.25) -> (-2.75, 2.75)
  point P0 (-18, 18)
  constraint coincident A2.centre L236.start
  constraint coincident A0.centre L236.end
  constraint coincident A3.centre L237.end
  constraint coincident A1.centre L238.end
  constraint midpoint L237 P0
extrude "Extrude3" [rolled back] along distance 1.5 taper angle 0

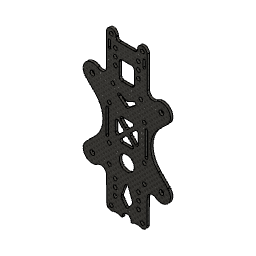
design "frame_main_2mm"
Autodesk Fusion 360 part; units mm, degrees
sketch "Sketch1" plane through (0, 0, 0) normal (0, 0, 1) x (1, 0, 0)